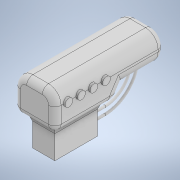
# Autodesk Inventor part: Weapon-Electric-Body
Saved by Autodesk Inventor 2020 (Build 240168000, 168)
## iProperties
Created: 2019-11-14
Part Number: Weapon-Electric-Body
Material: Generic
Document SubType Name: Modeling
Designer: vifly_01
Density: 1 g/cm^3
Appearance: Default
Author: vifly_01
Autodesk Inventor part; units mm, degrees
ref_plane "YZ Plane" through (0, 0, 0) normal (1, 0, 0) x (0, 1, 0)
ref_plane "XZ Plane" through (0, 0, 0) normal (0, 1, 0) x (-1, 0, 0)
ref_plane "XY Plane" through (0, 0, 0) normal (0, 0, 1) x (1, 0, 0)
sketch "Sketch1" plane through (0, 0, 0) normal (0, 0, 1) x (1, 0, 0)
  line L0 (6.5, -8.75) -> (-6.5, -8.75)
  line L1 (-6.5, -8.75) -> (-6.5, 8.75)
  line L2 (-6.5, 8.75) -> (6.5, 8.75)
  line L3 (6.5, 8.75) -> (6.5, -8.75)
  line L4 (6.5, -8.75) -> (-6.5, 8.75) construction
  line L5 (-6.5, -8.75) -> (6.5, 8.75) construction
  point P0 (0, 0)
  dimension "d0" = 13
  dimension "d1" = 17.5
  constraints: 12 end point, 2 midpoint, 2 parallel, 1 horizontal, 1 perpendicular
  measures "d0" distance of L1.end L2.end
  measures "d1" distance of L0.end L1.end
extrude "Extrusion1" add sketch "Sketch1" along normal blind 35
sketch "Sketch2" plane through (6.5, -8.75, 0) normal (1, 0, 0) x (0, 0, -1)
  line L0 (0, 0) -> (-35, 0) projected
  line L1 (-17.0033, 0) -> (-10.7814, 6.2327)
  line L2 (-10.7814, 6.2327) -> (0, 6.2327)
  line L3 (0, 6.2327) -> (0, 0)
  line L4 (0, 0) -> (-17.0033, 0)
  line L5 (-10.7814, 6.2327) -> (-35, 6.2327)
  line L6 (-35, 17.5) -> (-35, 0) projected
  line L7 (-35, 6.2327) -> (-35, 0)
  line L8 (-35, 0) -> (-17.0033, 0)
  point P0 (0, 8.75)
  constraints: 14 end point, 3 perpendicular, 1 collinear, 1 horizontal, 1 parallel, 1 point on line
extrude "Extrusion2" cut sketch "Sketch2" against normal blind 35
sketch "Sketch6" plane through (6.5, 8.75, 35) normal (1, 0, 0) x (0, 0, -1)
  line L0 (35, -8.75) -> (22.5, -8.75)
  line L1 (22.5, -8.75) -> (20.8857, -11.2673)
  line L2 (0, -11.2673) -> (35, -11.2673) projected
  line L3 (20.8857, -11.2673) -> (35, -11.2673)
  line L4 (35, -11.2673) -> (35, -8.75)
  line L5 (35, 0) -> (35, -11.2673) projected
  dimension "d21" = 12.5
  constraints: 8 end point, 2 horizontal, 1 collinear, 1 point on line
  measures "d21" distance of L0.start L0.end
extrude "Extrusion6" cut sketch "Sketch6" against normal blind 20
fillet "Fillet4" radius 4 4 edges at (6.5, 0, 6.25) (-6.5, 0, 6.25) (6.5, -1.2586, 13.3072) (-6.5, -1.2586, 13.3072)
fillet "Fillet5" radius 4 2 edges at (-6.5, 8.75, 17.5) (6.5, 8.75, 17.5)
fillet "Fillet6" radius 2 19 edges at (5.3284, -2.5173, 15.5061) (0, -2.5173, 14.1143) (-5.3284, -2.5173, 15.5061) (-6.5, -2.5173, 26.9331) (6.5, -2.5173, 26.9331) (5.3284, 7.5784, 35) (0, 8.75, 35) (-5.3284, 7.5784, 35) (-6.5, 1.1164, 35) (6.5, 1.1164, 35) (-5.3284, 7.5784, 0) (-6.5, 4.375, 0) (-5.3284, 1.1716, 0) (0, 0, 0) (5.3284, 1.1716, 0) (6.5, 4.375, 0) (5.3284, 7.5784, 0) (0, 8.75, 0) (0, -2.5173, 35)
sketch "Sketch7" plane through (-4.5, -2.5173, 33) normal (0, -1, 0) x (1, 0, 0)
  line L0 (9, 0) -> (9, -15.4164) projected
  line L1 (0, -15.4164) -> (0, 0) projected
  line L2 (9, 0) -> (0, 0)
  line L3 (0, 0) -> (0, -15.4164)
  line L4 (0, -15.4164) -> (9, -15.4164)
  line L5 (9, -15.4164) -> (9, 0)
  point P0 (4.5, -33)
  constraints: 8 end point, 2 parallel, 1 horizontal, 1 perpendicular
extrude "Extrusion7" add sketch "Sketch7" along normal blind 2.5 draft -20
sketch "Sketch8" plane through (-4.5, -5.0173, 33) normal (0, -1, 0) x (1, 0, 0)
  line L0 (0.9099, -0.9099) -> (8.0901, -0.9099) projected
  line L1 (0.9099, -14.5065) -> (0.9099, -0.9099) projected
  line L2 (8.0901, -0.9099) -> (0.9099, -0.9099)
  line L3 (0.9099, -0.9099) -> (0.9099, -14.5065)
  line L4 (0.9099, -14.5065) -> (8.0901, -14.5065)
  line L5 (8.0901, -14.5065) -> (8.0901, -0.9099)
  point P0 (4.5, -33)
  constraints: 8 end point, 2 parallel, 1 horizontal, 1 perpendicular
extrude "Extrusion8" add sketch "Sketch8" along normal blind 7.5
sketch "Sketch10" plane through (6.5, -0.5173, 33) normal (1, 0, 0) x (0, 0, -1)
  line L0 (31, 5.2673) -> (0, 5.2673) projected
  circle A0 centre (2, 5.2673) radius 1.25
  circle A1 centre (6, 5.2673) radius 1.25
  circle A2 centre (10, 5.2673) radius 1.25
  circle A3 centre (14, 5.2673) radius 1.25
  point P0 (33, 0.5173)
  dimension "d41" = 2.5
  dimension "d44" = 4
  constraints: 4 centre point, 1 horizontal, 1 point on line, 6 other
  measures "d41" diameter of A0
  measures "d44" distance of A0.centre A1.centre
extrude "Extrusion10" add sketch "Sketch10" along normal mid plane 1
sketch "Sketch12" plane through (0, 0, 0) normal (1, 0, 0) x (0, 1, 0)
  line L0 (0, 2) -> (-0.7398, 2)
  line L1 (0, 3.1186) -> (-1.1197, 3.1186)
  line L2 (-5.0173, 18.4935) -> (-12.5173, 18.4935) projected
  line L3 (-11.2714, 18.4935) -> (-11.2714, 12.5316)
  arc A0 (-11.2714, 12.5316) -> (-0.7398, 2) centre (-0.7398, 12.5316) ccw
  point P0 (0, 0)
  constraints: 6 end point, 2 horizontal, 2 point on circle, 2 tangent, 1 centre point, 1 point on line, 1 vertical
sketch "Sketch13" plane through (3.5901, -5.0173, 18.4935) normal (0, 0, -1) x (-1, 0, 0)
  circle A0 centre (3.5901, -3.9827) radius 0.375
  circle A1 centre (3.5901, -6.2631) radius 0.375
  point P0 (3.5901, 5.0173)
  dimension "d51" = 0.75
  dimension "d54" = 0.75
  dimension "d57" = 9
  dimension "d58" = 11.2804
  constraints: 2 centre point
  measures "d51" diameter of A0
  measures "d54" diameter of A1
  measures "d57" distance of A0.centre point (3.59, 5.017)
  measures "d58" distance of A1.centre point (3.59, 5.017)
sweep "Sweep2" add profiles "Sketch13" path "Sketch12" path curves L3 A0 L0
body "Solid1"
